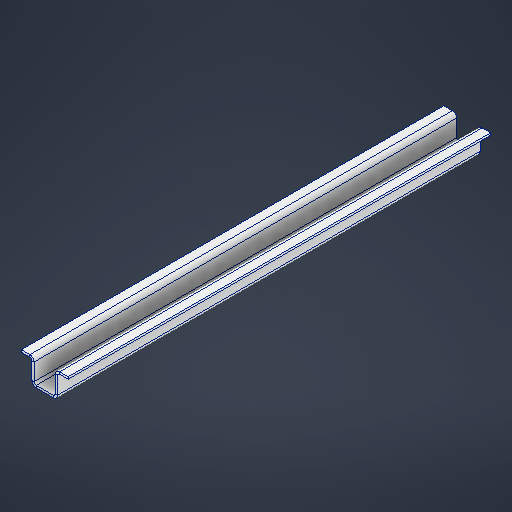
# Autodesk Inventor part: Stringer
Saved by Autodesk Inventor 2026.2 (Build 302298000, 298)
## iProperties
Created: 2026-02-13
Part Number: Stringer
Material: Aluminum 6061
Document SubType Name: Sheet Metal
Designer: Lex Machina
Density: 2.7 g/cm^3
Sheet Metal Rule: Default
Appearance: Aluminum - Flat
Mass: 346.725 g
Surface Area: 1057.31 cm^2
Volume: 128.417 cm^3
Author: Lex Machina
Autodesk Inventor part; units mm, degrees
ref_plane "YZ Plane" through (0, 0, 0) normal (1, 0, 0) x (0, 1, 0)
ref_plane "XZ Plane" through (0, 0, 0) normal (0, 1, 0) x (-1, 0, 0)
ref_plane "XY Plane" through (0, 0, 0) normal (0, 0, 1) x (1, 0, 0)
sketch "Sketch1" plane through (0, 0, 0) normal (0, 1, 0) x (-1, 0, 0)
  line L0 (0, 0) -> (30, 0)
  line L1 (30, 0) -> (30, -496)
  line L2 (30, -496) -> (0, -496)
  line L3 (0, -496) -> (0, 0)
  dimension "d0" = 30
  dimension "d1" = 496
  measures "d0" distance of L1.end L2.end
  measures "d1" distance of L0.end L1.end
extrude "Plate1" add sketch "Sketch1" along normal blind 2.5
sketch "Sketch2" plane through (-27.5, 0, 0) normal (-1, 0, 0) x (0, -1, 0)
  line L0 (0, -496) -> (0, 0)
  line L1 (0, 0) -> (-30, 0)
  line L2 (-30, 0) -> (-30, -496)
  line L3 (-30, -496) -> (0, -496)
  constraints: 6 end point, 1 horizontal, 1 perpendicular, 1 vertical
edge flange "Flange1" height 30 angle 90 thickness 2.5 bend radius 2.5 thickness toward (-1, 0, 0) relief straight relief width 2.5 relief depth 1.25 corner gap 2.5 corner form 0 edges at (-30, 2.5, -248) (0, 2.5, -248) wall of the first edge with corners at (-27.5, 0, -496) (-27.5, 0, 0) (-27.5, 30, 0) (-27.5, 30, -496)
bend "Bend1"
corner "Corner1"
sketch "Sketch3" plane through (-27.5, 27.5, -496) normal (0, 1, 0) x (-1, 0, 0)
  line L0 (0, 496) -> (0, 0)
  line L1 (0, 0) -> (15, 0)
  line L2 (15, 0) -> (15, 496)
  line L3 (15, 496) -> (0, 496)
  constraints: 6 end point, 1 horizontal, 1 perpendicular, 1 vertical
edge flange "Flange2" height 15 angle 90 thickness 2.5 bend radius 2.5 thickness toward (0, 1, 0) relief straight relief width 2.5 relief depth 1.25 corner gap 2.5 corner form 0 edges at (-30, 30, -248) (0, 30, -248) wall of the first edge with corners at (-27.5, 27.5, 0) (-27.5, 27.5, -496) (-42.5, 27.5, -496) (-42.5, 27.5, 0)
bend "Bend2"
corner "Corner2"
equation "\"d2\" = Thickness"
equation "\"d3\" = BendReliefWidth"
equation "\"d4\" = BendReliefDepth"
equation "\"d5\" = MinimumRemnant"
equation "\"d6\" = TransitionRadius"
equation "\"d9\" = BendRadius"
equation "\"d10\" = CornerReliefSize"
equation "\"d11\" = GapSize"
equation "\"d12\" = JacobiRadiusSize"
equation "\"d13\" = BendReliefWidth"
equation "\"d14\" = BendReliefDepth"
equation "\"d15\" = MinimumRemnant"
equation "\"d16\" = TransitionRadius"
equation "\"d19\" = BendRadius"
equation "\"d20\" = CornerReliefSize"
equation "\"d21\" = GapSize"
equation "\"d22\" = JacobiRadiusSize"
equation "\"BendRadius\" = Thickness"
equation "\"BendReliefWidth\" = Thickness"
equation "\"BendReliefDepth\" = 0.5 * Thickness"
equation "\"MinimumRemnant\" = 2 * Thickness"
equation "\"TransitionRadius\" = BendRadius"
equation "\"JacobiRadiusSize\" = BendRadius"
equation "\"GapSize\" = Thickness"
equation "\"Thickness\" = 2.5"
equation "\"CornerReliefSize\" = 10"
body "Solid1"
